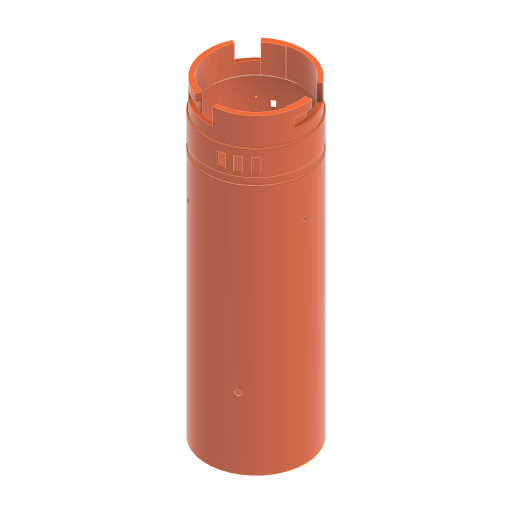
# Autodesk Inventor part: Lower skin
Saved by Autodesk Inventor 2024 (Build 280153000, 153)
## iProperties
Created: 2023-12-30
Part Number: Lower skin
Material: Plastic, Opaque White
Document SubType Name: Modeling
Designer: Jamie
Density: 0.952 g/cm^3
Appearance: Smooth - Light Orange
Author: Jamie
Autodesk Inventor part; units mm, degrees
ref_plane "XZ Plane" through (0, 0, 0) normal (0, 1, 0) x (-1, 0, 0)
ref_plane "XY Plane" through (0, 0, 0) normal (0, 0, 1) x (1, 0, 0)
sketch "Sketch1" plane through (0, 0, 0) normal (0, 1, 0) x (-1, 0, 0)
  circle A0 centre (0, 0) radius 35
  circle A1 centre (0, 0) radius 34.5
  dimension "d0" = 70
  dimension "d1" = 69
  constraints: 2 centre point, 2 coincident
  measures "d0" diameter of A0
  measures "d1" diameter of A1
extrude "Extrusion1" add sketch "Sketch1" along normal blind 200.5
ref_plane "Work Plane2" through (35, 0, 0) normal (1, 0, 0) x (0, 1, 0)
sketch "Sketch4" plane through (35, 0, 0) normal (1, 0, 0) x (0, 1, 0)
  line L0 (200.5, -35) -> (200.5, 35) projected
  point P0 (0, 0)
  point P1 (150.5, 0)
  dimension "d48" = 150.5
  measures "d48" distance of point (0, 0) point (150.5, 0)
hole "Hole2" at (35, 150.5, 0) direction (-1, 0, 0) diameter 3 depth 8 tip angle 118
sketch "Sketch5" plane through (0, 200.5, 0) normal (0, 1, 0) x (1, 0, 0)
  circle A0 centre (0, 0) radius 34
  circle A1 centre (0, 0) radius 31
  dimension "d44" = 68
  dimension "d45" = 62
  constraints: 2 centre point, 2 coincident
  measures "d44" diameter of A0
  measures "d45" diameter of A1
extrude "Extrusion3" add sketch "Sketch5" along normal blind 20
sketch "Sketch6" plane through (0, 200.5, 0) normal (0, -1, 0) x (1, 0, 0)
  circle A0 centre (0, 0) radius 33.5
  circle A1 centre (0, 0) radius 34.5 projected
  circle A2 centre (0, 0) radius 35
  constraints: 2 centre point, 2 coincident
extrude "Extrusion4" add sketch "Sketch6" along normal blind 27.5 contours A1
ref_plane "Work Plane4" through (34, 0, 0) normal (1, 0, 0) x (0, 1, 0)
sketch "Sketch9" plane through (0, 0, 0) normal (0, -1, 0) x (1, 0, 0)
  line L0 (34.2575, 0) -> (34.2575, -4.0836) construction
  circle A0 centre (0, 0) radius 31 projected
  line L1 (0, 0) -> (30.529, -5.3831) construction
  line L2 (0, 0) -> (31, 0) construction
  line L3 (30.529, -5.3831) -> (34.2575, -6.0405)
  line L4 (30.529, -5.3831) -> (34.5805, -2.5462)
  line L5 (34.2575, -6.0405) -> (34.5805, -2.5462)
  point P0 (30.5793, -5.0896)
  point P1 (30.529, -5.3831)
  dimension "d73" = 0
  dimension "d81" = 10
  dimension "d83" = 45
  constraints: 12 end point, 3 point on circle, 1 coincident, 1 horizontal, 1 vertical
  measures "d73" vertical distance of point (0, 0) L0.start
  measures "d81" angle of L2 L1
  measures "d83" angle of L1 L4
extrude "Extrusion5" add sketch "Sketch9" against normal blind 30 contours L4 L5 L3
mirror "Mirror1" about plane through (0, 0, 0) normal (0, 0, 1) of "Extrusion5"
pattern_circular "Circular Pattern4" count 3 over 360 about axis through (0, 0, 0) along (0, 1, 0) of "Hole2"
ref_plane "Work Plane5" through (0, 212.75, 0) normal (0, 1, 0) x (1, 0, 0)
sketch "Sketch10" plane through (0, 212.75, 0) normal (0, 1, 0) x (1, 0, 0)
  circle A0 centre (0, 0) radius 31 projected
  line L0 (0, 0) -> (-17.0553, 29.5407) construction
  line L1 (-11.7997, 32.4194) -> (-10.6026, 29.1305) construction
  circle A1 centre (0, 0) radius 34 construction
  line L2 (0, 0) -> (-13.3331, 37.6515)
  line L3 (0, 0) -> (-27.0667, 31.6911)
  line L4 (-27.0667, 31.6911) -> (-13.3331, 37.6515)
  dimension "d88" = 10
  dimension "d90" = 10.5
  dimension "d93" = 21
  constraints: 8 end point, 1 other
  measures "d88" angle of L1 L0
  measures "d90" angle of L0 L2
  measures "d93" angle of L3 L2
extrude "Extrusion6" cut sketch "Sketch10" against normal blind 4.5 contours L2 L3 A0 | A0 L3 L4 L2 picked at (-10.3141, 17.8645)
sketch "Sketch11" plane through (0, 208.25, 0) normal (0, 1, 0) x (1, 0, 0)
  arc A0 (-11.3494, 32.0498) -> (-22.0812, 25.8538) centre (0, 0) ccw projected
  point P0 (-29.8798, 16.2234)
sketch "Sketch12" plane through (0, 208.25, 0) normal (0, 1, 0) x (1, 0, 0)
  line L0 (-22.0812, 25.8538) -> (0, 0)
  line L1 (0, 0) -> (-37.5141, 17.0962)
  line L2 (-37.5141, 17.0962) -> (-24.2656, 28.4114)
  line L3 (-24.2656, 28.4114) -> (-22.0812, 25.8538)
  dimension "d94" = 25
  constraints: 8 end point, 1 collinear, 1 perpendicular, 1 point on line
  measures "d94" angle of L1 L0
extrude "Extrusion7" cut sketch "Sketch12" along normal through all
pattern_circular "Circular Pattern5" count 3 over 360 about axis through (0, 200.5, 0) along (0, 1, 0) of "Extrusion6", "Extrusion7"
sketch "Sketch14" plane through (0, 200.5, 0) normal (0, -1, 0) x (1, 0, 0)
  arc A0 (-20.1329, -23.5726) -> (25.2376, -18.0018) centre (0, 0) ccw projected
  arc A1 (-20.1329, -23.5726) -> (-8.2844, -29.8725) centre (0, 0) ccw
  line L0 (-20.1329, -23.5726) -> (0, 0) construction
  line L1 (0, 0) -> (-8.2844, -29.8725) construction
  line L2 (-20.1329, -23.5726) -> (-19.4834, -22.8122)
  line L3 (-8.2844, -29.8725) -> (-7.5908, -27.3714)
  arc A2 (-19.4834, -22.8122) -> (-8.0172, -28.9089) centre (0, 0) ccw
  dimension "d102" = 25
  dimension "d103" = 30
  constraints: 8 end point, 5 point on circle, 3 point on line, 2 centre point, 2 coincident
  measures "d102" angle of L0 L1
  measures "d103" radius of A2
extrude "Extrusion8" add sketch "Sketch14" against normal blind 20
pattern_circular "Circular Pattern6" count 3 over 360 about axis through (0, 0, 0) along (0, 1, 0) of "Extrusion8"
chamfer "Chamfer1" distance 3 angle 45 1 edges at (-33.5, 200.5, 0)
sketch "Sketch16" plane through (0, 212.75, 0) normal (0, -1, 0) x (0.8660254, 0, 0.5)
  arc A0 (6.196, 33.4307) -> (-6.196, 33.4307) centre (0, 0) ccw projected
  line L0 (-5.6493, 30.4809) -> (-6.196, 33.4307) projected
  arc A1 (6.196, 33.4307) -> (-6.196, 33.4307) centre (0, 0) ccw
  line L1 (6.196, 33.4307) -> (5.6493, 30.4809) projected
  arc A2 (5.6493, 30.4809) -> (-5.6493, 30.4809) centre (0, 0) ccw projected
  arc A3 (5.6493, 30.4809) -> (-5.6493, 30.4809) centre (0, 0) ccw
  line L2 (5.6493, 30.4809) -> (6.196, 33.4307)
  line L3 (-5.6493, 30.4809) -> (-6.196, 33.4307)
  constraints: 4 end point, 4 point on circle, 2 centre point, 2 collinear
extrude "Extrusion9" cut sketch "Sketch16" against normal blind 2
pattern_circular "Circular Pattern7" count 3 over 360 about axis through (0, 0, 0) along (0, 1, 0) of "Extrusion9"
chamfer "Chamfer4" distance 12 angle 15 1 edges at (32.2525, 30, 5.687) measured on face at (32.2525, 29.5, 5.687)
chamfer "Chamfer5" distance 12 angle 15 1 edges at (32.2525, 30, -5.687) measured on face at (32.2525, 29.5, -5.687)
pattern_circular "Circular Pattern8" count 3 over 360 about axis through (0, 0, 0) along (0, 1, 0) of "Extrusion5", "Mirror1", "Chamfer4", "Chamfer5"
chamfer "Chamfer6" distance 1 angle 45 1 edges at (-33.5, 173, 0)
sketch "Sketch17" plane through (35, 0, 0) normal (1, 0, 0) x (0, 1, 0)
  point P0 (0, 0)
ref_plane "Work Plane6" through (30.529, 0, 5.3831) normal (-0.5, 0, -0.8660254) x (0, 1, 0)
sketch "Sketch18" plane through (30.529, 0, 5.3831) normal (-0.5, 0, -0.8660254) x (0, 1, 0)
  line L0 (0, 2.6812) -> (0, -50.1759) projected
  point P0 (0, -23.7474)
  point P1 (50, -23.7474)
  point P2 (0, -23.7474)
  dimension "d136" = 50
  constraints: 1 midpoint
  measures "d136" distance of point (0, -23.747) point (50, -23.747)
hole "Hole5" at (9.9632, 50, 17.2568) direction (0.5, 0, 0.8660254) diameter 4 depth 23.25 tip angle 118
sketch "Sketch19" plane through (30.529, 0, 5.3831) normal (-0.5, 0, -0.8660254) x (0, 1, 0)
  line L0 (195.5, -21.2474) -> (185.5, -21.2474)
  line L1 (185.5, -21.2474) -> (185.5, -26.2474)
  line L2 (185.5, -26.2474) -> (195.5, -26.2474)
  line L3 (195.5, -26.2474) -> (195.5, -21.2474)
  line L4 (220.5, -37.8469) -> (220.5, 8.3024) projected
  point P0 (0, -23.7474)
  point P1 (195.5, -23.7474)
  point P2 (149, -23.7474)
  dimension "d144" = 10
  dimension "d145" = 5
  dimension "d146" = 25
  dimension "d147" = 2.5
  constraints: 8 end point, 2 parallel, 1 horizontal, 1 midpoint, 1 perpendicular
  measures "d144" distance of L0.start L0.end
  measures "d145" distance of L2.end L0.start
  measures "d146" distance from line of L4 point (195.5, -23.747)
  measures "d147" distance from line of L0 point (149, -23.747)
extrude "Extrusion10" cut sketch "Sketch19" against normal blind 200.5
pattern_circular "Circular Pattern9" count 2 over 15 about axis through (0, 0, 0) along (0, 1, 0) of "Extrusion10"
pattern_circular "Circular Pattern10" count 2 over 15 about axis through (0, 0, 0) along (0, -1, 0) of "Extrusion10"
sketch "Sketch20" plane through (30.529, 0, 5.3831) normal (-0.5, 0, -0.8660254) x (0, 1, 0)
  line L0 (178, -22.2474) -> (183, -22.2474)
  line L1 (183, -22.2474) -> (183, -25.2474)
  line L2 (183, -25.2474) -> (178, -25.2474)
  line L3 (178, -25.2474) -> (178, -22.2474)
  line L4 (195.5, -21.2474) -> (185.5, -21.2474) projected
  line L5 (185.5, -21.2474) -> (185.5, -26.2474) projected
  line L6 (195.5, -26.2474) -> (195.5, -21.2474) projected
  point P0 (0, -23.7474)
  point P1 (180.5, -25.2474)
  dimension "d160" = 3
  dimension "d161" = 1
  dimension "d162" = 5
  dimension "d168" = 12.5
  constraints: 8 end point, 2 parallel, 1 horizontal, 1 midpoint, 1 perpendicular
  measures "d160" distance from line of point (180.5, -25.247) L0
  measures "d161" distance between parallel lines of L4 L0
  measures "d162" distance between parallel lines of L1 L3
  measures "d168" distance between parallel lines of L1 L6
extrude "Extrusion11" cut sketch "Sketch20" along normal blind 200.5
sketch "Sketch21" plane through (0, 183, 0) normal (0, -1, 0) x (0.8660254, 0, -0.5)
  circle A0 centre (0, 0) radius 44.2467
  circle A1 centre (0, 0) radius 34.5
  constraints: 2 centre point, 2 coincident
extrude "Extrusion12" cut sketch "Sketch21" along normal blind 5
body "Solid1"
